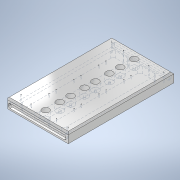
# Autodesk Inventor part: Assembly Plate
Saved by Autodesk Inventor 2022 (Build 260153000, 153)
## iProperties
Created: 2022-03-23
Part Number: Assembly Plate
Material: Generic
Document SubType Name: Modeling
Designer: Caleb
Density: 1 g/cm^3
Appearance: Aluminum - Dark
Author: Caleb
Autodesk Inventor part; units mm, degrees
ref_plane "YZ Plane" through (0, 0, 0) normal (1, 0, 0) x (0, 1, 0)
ref_plane "XZ Plane" through (0, 0, 0) normal (0, 1, 0) x (-1, 0, 0)
ref_plane "XY Plane" through (0, 0, 0) normal (0, 0, 1) x (1, 0, 0)
sketch "Sketch1" plane through (0, 0, 0) normal (0, 1, 0) x (-1, 0, 0)
  line L0 (-63.5, -107.95) -> (63.5, -107.95)
  line L1 (63.5, -107.95) -> (63.5, 107.95)
  line L2 (63.5, 107.95) -> (-63.5, 107.95)
  line L3 (-63.5, 107.95) -> (-63.5, -107.95)
  line L4 (-63.5, -107.95) -> (63.5, 107.95) construction
  line L5 (63.5, -107.95) -> (-63.5, 107.95) construction
  point P0 (0, 0)
  dimension "d0" = 127
  dimension "d1" = 215.9
  constraints: 12 end point, 2 midpoint, 2 parallel, 1 horizontal, 1 perpendicular
  measures "d0" distance of L2.end L1.end
  measures "d1" distance of L1.end L0.end
extrude "Extrusion1" add sketch "Sketch1" along normal blind 19.05
sketch "Sketch4" plane through (0, 19.05, 0) normal (0, 1, 0) x (1, 0, 0)
  line L0 (-63.5, -107.95) -> (63.5, -107.95) projected
  line L1 (-63.5, 107.95) -> (-63.5, -107.95) projected
  point P0 (0, 0)
  point P1 (0, -90.5002)
  point P2 (0, -61.8871)
  point P3 (0, -11.0871)
  point P4 (0, -39.7002)
  point P5 (0, 39.7129)
  point P6 (0, 11.0998)
  point P7 (0, 90.5129)
  point P8 (0, 61.8998)
  dimension "d14" = 17.4498
  dimension "d15" = 46.0629
  dimension "d18" = 50.8
  constraints: 1 vertical, 6 other
  measures "d14" distance from line of L0 point (0, -90.5)
  measures "d15" distance from line of L0 point (0, -61.887)
  measures "d18" distance of point (0, -61.887) point (0, -11.087)
hole "Hole2" at (0, 19.05, 90.5002) at (0, 19.05, 61.8871) at (0, 19.05, 11.0871) at (0, 19.05, 39.7002) at (0, 19.05, -39.7129) at (0, 19.05, -11.0998) at (0, 19.05, -90.5129) at (0, 19.05, -61.8998) direction (0, -1, 0) diameter 3.9624 end through all counterbore diameter 13.97 counterbore depth 15.24 thread size "10-32 UNF" class "2B" standard "ANSI Unified Screw Threads"
sketch "Sketch5" plane through (0, 19.05, 0) normal (0, 1, 0) x (1, 0, 0)
  line L0 (-63.5, -107.95) -> (63.5, -107.95) projected
  line L1 (63.5, 107.95) -> (-63.5, 107.95) projected
  line L2 (-63.5, 107.95) -> (-63.5, -107.95) projected
  line L3 (63.5, -107.95) -> (63.5, 107.95) projected
  point P0 (0, 0)
  point P1 (-53.15, -87.9)
  point P2 (-53.15, 97.6)
  point P3 (53.15, 97.6)
  point P4 (53.15, -97.6)
  dimension "d31" = 20.05
  dimension "d32" = 10.35
  dimension "d33" = 10.35
  dimension "d34" = 10.35
  dimension "d35" = 10.35
  dimension "d36" = 10.35
  dimension "d37" = 10.35
  dimension "d38" = 10.35
  measures "d31" distance from line of L0 point (-53.15, -87.9)
  measures "d32" distance from line of L0 point (53.15, -97.6)
  measures "d33" distance from line of L1 point (53.15, 97.6)
  measures "d34" distance from line of L1 point (-53.15, 97.6)
  measures "d35" distance from line of L2 point (-53.15, 97.6)
  measures "d36" distance from line of L3 point (53.15, 97.6)
  measures "d37" distance from line of L3 point (53.15, -97.6)
  measures "d38" distance from line of L2 point (-53.15, -87.9)
hole "Hole3" at (-53.15, 19.05, 87.9) at (-53.15, 19.05, -97.6) at (53.15, 19.05, -97.6) at (53.15, 19.05, 97.6) direction (0, -1, 0) diameter 1.0211 end through all thread size "00-96 NS" class "2B" standard "ANSI Unified Screw Threads"
sketch "Sketch6" plane through (0, 19.05, 0) normal (0, 1, 0) x (1, 0, 0)
  line L0 (-63.5, -107.95) -> (63.5, -107.95) projected
  line L1 (-63.5, 107.95) -> (-63.5, -107.95) projected
  point P0 (0, 0)
  point P1 (-25.75, -94.25)
  point P2 (-25.75, -58.15)
  point P3 (25.75, -58.15)
  point P4 (25.75, -94.25)
  point P5 (25.75, -43.45)
  point P6 (25.75, -7.35)
  point P7 (-25.75, -7.35)
  point P8 (-25.75, -43.45)
  point P9 (25.75, 7.35)
  point P10 (25.75, 43.45)
  point P11 (-25.75, 43.45)
  point P12 (-25.75, 7.35)
  point P13 (25.75, 58.15)
  point P14 (25.75, 94.25)
  point P15 (-25.75, 94.25)
  point P16 (-25.75, 58.15)
  dimension "d46" = 36.1
  dimension "d47" = 51.5
  dimension "d48" = 13.7
  dimension "d49" = 37.75
  dimension "d52" = 50.8
  constraints: 2 horizontal alignment, 2 vertical alignment, 1 vertical, 12 other
  measures "d46" distance of point (-25.75, -58.15) point (-25.75, -94.25)
  measures "d47" distance of point (25.75, -94.25) point (-25.75, -94.25)
  measures "d48" distance from line of L0 point (-25.75, -94.25)
  measures "d49" distance from line of L1 point (-25.75, -94.25)
  measures "d52" distance of point (25.75, -94.25) point (25.75, -43.45)
hole "Hole4" at (-25.75, 19.05, 94.25) at (-25.75, 19.05, 58.15) at (25.75, 19.05, 58.15) at (25.75, 19.05, 94.25) at (25.75, 19.05, 43.45) at (25.75, 19.05, 7.35) at (-25.75, 19.05, 7.35) at (-25.75, 19.05, 43.45) at (25.75, 19.05, -7.35) at (25.75, 19.05, -43.45) at (-25.75, 19.05, -43.45) at (-25.75, 19.05, -7.35) at (25.75, 19.05, -58.15) at (25.75, 19.05, -94.25) at (-25.75, 19.05, -94.25) at (-25.75, 19.05, -58.15) direction (0, -1, 0) diameter 1.1811 end through all thread size "0-80 UNF" class "2B" standard "ANSI Unified Screw Threads"
chamfer "Chamfer1" distance 3.175 angle 45 2 edges at (0, 19.05, 107.95) (63.5, 19.05, 0)
chamfer "Chamfer2" distance 3.175 angle 45 3 edges at (-1.5875, 19.05, -107.95) (-63.5, 19.05, -1.5875) (-63.5, 7.9375, 107.95)
sketch "Sketch7" plane through (0, 0, 0) normal (0, -1, 0) x (1, 0, 0)
  line L0 (15, 98.425) -> (39.45, 98.425)
  line L1 (44.45, 93.425) -> (44.45, -87.075)
  line L2 (39.45, -92.075) -> (15, -92.075)
  line L3 (10, -87.075) -> (10, 93.425)
  line L4 (63.5, 107.95) -> (63.5, -107.95) projected
  line L5 (-60.325, 107.95) -> (63.5, 107.95) projected
  line L6 (63.5, -107.95) -> (-63.5, -107.95) projected
  circle A0 centre (0, 90.5002) radius 1.9812 projected
  arc A1 (15, 98.425) -> (10, 93.425) centre (15, 93.425) ccw
  arc A2 (44.45, 93.425) -> (39.45, 98.425) centre (39.45, 93.425) ccw
  arc A3 (39.45, -92.075) -> (44.45, -87.075) centre (39.45, -87.075) ccw
  arc A4 (10, -87.075) -> (15, -92.075) centre (15, -87.075) ccw
  line L7 (-60.325, 107.95) -> (63.5, 107.95) construction
  line L8 (0, 107.95) -> (0, -107.95) construction
  line L9 (-15, 98.425) -> (-39.45, 98.425)
  line L10 (-44.45, 93.425) -> (-44.45, -87.075)
  line L11 (-39.45, -92.075) -> (-15, -92.075)
  line L12 (-10, -87.075) -> (-10, 93.425)
  arc A5 (-10, 93.425) -> (-15, 98.425) centre (-15, 93.425) ccw
  arc A6 (-39.45, 98.425) -> (-44.45, 93.425) centre (-39.45, 93.425) ccw
  arc A7 (-44.45, -87.075) -> (-39.45, -92.075) centre (-39.45, -87.075) ccw
  arc A8 (-15, -92.075) -> (-10, -87.075) centre (-15, -87.075) ccw
  point P0 (0, 0)
  dimension "d70" = 19.05
  dimension "d71" = 9.525
  dimension "d72" = 15.875
  dimension "d73" = 10
  dimension "d74" = 5
  constraints: 18 end point, 16 point on circle, 12 symmetric about line, 8 centre point, 8 tangent, 3 equal radius, 2 parallel, 1 horizontal, 1 midpoint, 1 perpendicular, 1 point on line, 4 other
  measures "d70" distance between parallel lines of L4 L1
  measures "d71" distance between parallel lines of L5 L0
  measures "d72" distance between parallel lines of L6 L2
  measures "d73" distance from line of L3 A0.centre
  measures "d74" radius of A1
extrude "Extrusion3" cut sketch "Sketch7" against normal blind 12.7 contours L0 A2 L1 A3 L2 A4 L3 A1 | A5 L12 A8 L11 A7 L10 A6 L9
sketch "Sketch8" plane through (63.5, 0, -107.95) normal (0, 0, -1) x (-1, 0, 0)
  line L0 (119.0625, 3.175) -> (7.9375, 3.175)
  line L1 (4.7625, 6.35) -> (4.7625, 8.89)
  line L2 (7.9375, 12.065) -> (119.0625, 12.065)
  line L3 (122.2375, 8.89) -> (122.2375, 6.35)
  line L4 (122.2375, 3.175) -> (4.7625, 12.065) construction
  line L5 (4.7625, 3.175) -> (122.2375, 12.065) construction
  line L6 (0, 0) -> (0, 15.875) projected
  line L7 (127, 0) -> (127, 15.875) projected
  line L8 (0, 0) -> (127, 0) projected
  arc A0 (7.9375, 12.065) -> (4.7625, 8.89) centre (7.9375, 8.89) ccw
  arc A1 (4.7625, 6.35) -> (7.9375, 3.175) centre (7.9375, 6.35) ccw
  arc A2 (119.0625, 3.175) -> (122.2375, 6.35) centre (119.0625, 6.35) ccw
  arc A3 (122.2375, 8.89) -> (119.0625, 12.065) centre (119.0625, 8.89) ccw
  point P0 (63.5, 0)
  point P1 (63.5, 7.62)
  dimension "d77" = 8.89
  dimension "d78" = 4.7625
  dimension "d79" = 4.7625
  dimension "d80" = 3.175
  dimension "d83" = 3.175
  constraints: 12 end point, 8 point on circle, 8 point on line, 8 tangent, 4 centre point, 3 equal radius, 2 midpoint, 2 parallel, 1 horizontal, 1 perpendicular
  measures "d77" distance of L5.start L4.end
  measures "d78" distance between parallel lines of L6 L1
  measures "d79" distance between parallel lines of L7 L3
  measures "d80" distance between parallel lines of L8 L0
  measures "d83" radius of A0
extrude "Extrusion4" cut sketch "Sketch8" against normal blind 4.7625
sketch "Sketch9" plane through (63.5, 0, 107.95) normal (0, 0, 1) x (1, 0, 0)
  line L0 (-7.9375, 3.175) -> (-119.0625, 3.175)
  line L1 (-122.2375, 6.35) -> (-122.2375, 8.89)
  line L2 (-119.0625, 12.065) -> (-7.9375, 12.065)
  line L3 (-4.7625, 8.89) -> (-4.7625, 6.35)
  line L4 (-4.7625, 3.175) -> (-122.2375, 12.065) construction
  line L5 (-122.2375, 3.175) -> (-4.7625, 12.065) construction
  arc A0 (-119.0625, 12.065) -> (-122.2375, 8.89) centre (-119.0625, 8.89) ccw
  arc A1 (-122.2375, 6.35) -> (-119.0625, 3.175) centre (-119.0625, 6.35) ccw
  arc A2 (-7.9375, 3.175) -> (-4.7625, 6.35) centre (-7.9375, 6.35) ccw
  arc A3 (-4.7625, 8.89) -> (-7.9375, 12.065) centre (-7.9375, 8.89) ccw
  line L6 (-123.825, 0) -> (0, 0) projected
  line L7 (-127, 15.875) -> (-127, 0) projected
  point P0 (63.5, 0)
  point P1 (-63.5, 7.62)
  dimension "d84" = 8.89
  dimension "d88" = 3.175
  dimension "d89" = 3.175
  dimension "d90" = 4.7625
  constraints: 12 end point, 8 point on circle, 8 point on line, 8 tangent, 4 centre point, 3 equal radius, 2 midpoint, 2 parallel, 1 horizontal, 1 perpendicular
  measures "d84" distance of L5.start L4.end
  measures "d88" radius of A0
  measures "d89" distance between parallel lines of L6 L0
  measures "d90" distance between parallel lines of L7 L1
extrude "Extrusion5" cut sketch "Sketch9" against normal blind 4.7625
equation "\"d79\" = d78"
body "Solid1"
